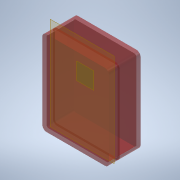
# Autodesk Inventor part: bottom
Saved by Autodesk Inventor 2020 (Build 240168000, 168)
## iProperties
Created: 2019-03-25
Part Number: bottom
Material: Generic
Document SubType Name: Modeling
Designer: erwin
Density: 1 g/cm^3
Appearance: Default
Author: erwin
Autodesk Inventor part; units mm, degrees
ref_plane "YZ Plane" through (0, 0, 0) normal (1, 0, 0) x (0, 1, 0)
ref_plane "XZ Plane" through (0, 0, 0) normal (0, 1, 0) x (-1, 0, 0)
ref_plane "Work Plane3" through (-33.721, -16.0631, -8.3772) normal (0, 0, -1) x (-1, 0, 0)
sketch "Sketch2" plane through (-33.721, -16.0631, -8.3772) normal (0, 0, -1) x (-1, 0, 0)
  line L0 (3.351, 52.725) -> (-59.649, 52.725)
  line L1 (-59.649, 52.725) -> (-59.649, -27.275)
  line L2 (-59.649, -27.275) -> (3.351, -27.275)
  line L3 (3.351, -27.275) -> (3.351, 52.725)
  line L4 (3.351, 52.725) -> (-59.649, -27.275) construction
  line L5 (-59.649, 52.725) -> (3.351, -27.275) construction
  line L6 (-25.524, -24.775) -> (-3.524, -24.775) projected
  line L7 (-0.024, 32.975) -> (-0.024, 14.6) projected
  line L8 (-56.274, -10.275) -> (-56.274, 32.975)
  line L9 (-3.524, 50.225) -> (-25.524, 50.225) projected
  line L10 (-1.524, 34.475) -> (-56.274, 34.475) projected
  line L11 (-56.274, -11.775) -> (-56.274, 34.475) projected
  line L12 (-56.274, -11.775) -> (-1.524, -11.775) projected
  line L13 (-1.524, -11.775) -> (-1.1358, -11.7239) projected
  line L14 (-0.774, -11.574) -> (-1.1358, -11.7239) projected
  line L15 (-0.4633, -11.3357) -> (-0.774, -11.574) projected
  line L16 (-0.4633, -11.3357) -> (-0.225, -11.025) projected
  line L17 (-0.0751, -10.6632) -> (-0.225, -11.025) projected
  line L18 (-0.024, -10.275) -> (-0.0751, -10.6632) projected
  line L19 (-0.024, 0) -> (-0.024, -10.275) projected
  line L20 (-0.024, 0) -> (-14.65, 0) projected
  line L21 (-14.65, 14.6) -> (-14.65, 0) projected
  line L22 (-0.024, 14.6) -> (-14.65, 14.6) projected
  line L23 (-0.024, 32.975) -> (-0.024, 14.6) projected
  line L24 (-0.024, 32.975) -> (-0.0751, 33.3632) projected
  line L25 (-0.0751, 33.3632) -> (-0.225, 33.725) projected
  line L26 (-0.225, 33.725) -> (-0.4633, 34.0357) projected
  line L27 (-0.774, 34.274) -> (-0.4633, 34.0357) projected
  line L28 (-1.1358, 34.4239) -> (-0.774, 34.274) projected
  line L29 (-1.1358, 34.4239) -> (-1.524, 34.475) projected
  line L30 (-46.714, -1.95) -> (-47.364, -1.95) projected
  line L31 (-46.714, -1.95) -> (-46.714, -2.6) projected
  line L32 (-47.364, -2.6) -> (-46.714, -2.6) projected
  line L33 (-47.364, -2.6) -> (-47.364, -1.95) projected
  line L34 (-37.794, -7.64) -> (-38.444, -7.64) projected
  line L35 (-37.794, -8.29) -> (-37.794, -7.64) projected
  line L36 (-38.444, -8.29) -> (-37.794, -8.29) projected
  line L37 (-38.444, -8.29) -> (-38.444, -7.64) projected
  line L38 (-2.8885, -10.3772) -> (-3.149, -10.4) projected
  line L39 (-3.4095, -10.3772) -> (-3.149, -10.4) projected
  line L40 (-3.662, -10.3095) -> (-3.4095, -10.3772) projected
  line L41 (-3.899, -10.199) -> (-3.662, -10.3095) projected
  line L42 (-3.899, -10.199) -> (-4.1132, -10.0491) projected
  line L43 (-4.1132, -10.0491) -> (-4.2981, -9.8642) projected
  line L44 (-4.2981, -9.8642) -> (-4.448, -9.65) projected
  line L45 (-4.5585, -9.413) -> (-4.448, -9.65) projected
  line L46 (-4.5585, -9.413) -> (-4.6262, -9.1605) projected
  line L47 (-4.6262, -9.1605) -> (-4.649, -8.9) projected
  line L48 (-4.649, -8.9) -> (-4.6262, -8.6395) projected
  line L49 (-4.5585, -8.387) -> (-4.6262, -8.6395) projected
  line L50 (-4.5585, -8.387) -> (-4.448, -8.15) projected
  line L51 (-4.448, -8.15) -> (-4.2981, -7.9358) projected
  line L52 (-4.2981, -7.9358) -> (-4.1132, -7.7509) projected
  line L53 (-3.899, -7.601) -> (-4.1132, -7.7509) projected
  line L54 (-3.662, -7.4905) -> (-3.899, -7.601) projected
  line L55 (-3.662, -7.4905) -> (-3.4095, -7.4228) projected
  line L56 (-3.4095, -7.4228) -> (-3.149, -7.4) projected
  line L57 (-2.8885, -7.4228) -> (-3.149, -7.4) projected
  line L58 (-2.636, -7.4905) -> (-2.8885, -7.4228) projected
  line L59 (-2.399, -7.601) -> (-2.636, -7.4905) projected
  line L60 (-2.399, -7.601) -> (-2.1848, -7.7509) projected
  line L61 (-1.9999, -7.9358) -> (-2.1848, -7.7509) projected
  line L62 (-1.85, -8.15) -> (-1.9999, -7.9358) projected
  line L63 (-1.85, -8.15) -> (-1.7395, -8.387) projected
  line L64 (-1.7395, -8.387) -> (-1.6718, -8.6395) projected
  line L65 (-1.6718, -8.6395) -> (-1.649, -8.9) projected
  line L66 (-1.649, -8.9) -> (-1.6718, -9.1605) projected
  line L67 (-1.7395, -9.413) -> (-1.6718, -9.1605) projected
  line L68 (-1.7395, -9.413) -> (-1.85, -9.65) projected
  line L69 (-1.9999, -9.8642) -> (-1.85, -9.65) projected
  line L70 (-1.9999, -9.8642) -> (-2.1848, -10.0491) projected
  line L71 (-2.399, -10.199) -> (-2.1848, -10.0491) projected
  line L72 (-2.636, -10.3095) -> (-2.399, -10.199) projected
  line L73 (-2.636, -10.3095) -> (-2.8885, -10.3772) projected
  line L74 (-7.964, -8.29) -> (-7.314, -8.29) projected
  line L75 (-7.964, -8.29) -> (-7.964, -7.64) projected
  line L76 (-7.964, -7.64) -> (-7.314, -7.64) projected
  line L77 (-7.314, -7.64) -> (-7.314, -8.29) projected
  line L78 (-10.504, -10.83) -> (-9.854, -10.83) projected
  line L79 (-10.504, -10.18) -> (-10.504, -10.83) projected
  line L80 (-10.504, -10.18) -> (-9.854, -10.18) projected
  line L81 (-9.854, -10.18) -> (-9.854, -10.83) projected
  line L82 (-15.584, -10.83) -> (-14.934, -10.83) projected
  line L83 (-15.584, -10.18) -> (-15.584, -10.83) projected
  line L84 (-14.934, -10.18) -> (-15.584, -10.18) projected
  line L85 (-14.934, -10.18) -> (-14.934, -10.83) projected
  line L86 (-15.584, -8.29) -> (-14.934, -8.29) projected
  line L87 (-15.584, -7.64) -> (-15.584, -8.29) projected
  line L88 (-15.584, -7.64) -> (-14.934, -7.64) projected
  line L89 (-14.934, -7.64) -> (-14.934, -8.29) projected
  line L90 (-17.474, -7.64) -> (-17.474, -8.29) projected
  line L91 (-18.124, -8.29) -> (-17.474, -8.29) projected
  line L92 (-18.124, -7.64) -> (-18.124, -8.29) projected
  line L93 (-17.474, -7.64) -> (-18.124, -7.64) projected
  line L94 (-20.014, -7.64) -> (-20.014, -8.29) projected
  line L95 (-20.664, -8.29) -> (-20.014, -8.29) projected
  line L96 (-20.664, -7.64) -> (-20.664, -8.29) projected
  line L97 (-20.014, -7.64) -> (-20.664, -7.64) projected
  line L98 (-22.554, -7.64) -> (-22.554, -8.29) projected
  line L99 (-23.204, -8.29) -> (-22.554, -8.29) projected
  line L100 (-23.204, -7.64) -> (-23.204, -8.29) projected
  line L101 (-22.554, -7.64) -> (-23.204, -7.64) projected
  line L102 (-25.094, -7.64) -> (-25.094, -8.29) projected
  line L103 (-25.744, -8.29) -> (-25.094, -8.29) projected
  line L104 (-25.744, -7.64) -> (-25.744, -8.29) projected
  line L105 (-25.094, -7.64) -> (-25.744, -7.64) projected
  line L106 (-27.634, -7.64) -> (-27.634, -8.29) projected
  line L107 (-28.284, -8.29) -> (-27.634, -8.29) projected
  line L108 (-28.284, -8.29) -> (-28.284, -7.64) projected
  line L109 (-27.634, -7.64) -> (-28.284, -7.64) projected
  line L110 (-30.824, -10.83) -> (-30.174, -10.83) projected
  line L111 (-30.824, -10.18) -> (-30.824, -10.83) projected
  line L112 (-30.174, -10.18) -> (-30.824, -10.18) projected
  line L113 (-30.174, -10.18) -> (-30.174, -10.83) projected
  line L114 (-33.364, -10.83) -> (-32.714, -10.83) projected
  line L115 (-33.364, -10.18) -> (-33.364, -10.83) projected
  line L116 (-32.714, -10.18) -> (-33.364, -10.18) projected
  line L117 (-32.714, -10.18) -> (-32.714, -10.83) projected
  line L118 (-35.904, -10.83) -> (-35.254, -10.83) projected
  line L119 (-35.904, -10.18) -> (-35.904, -10.83) projected
  line L120 (-35.254, -10.18) -> (-35.904, -10.18) projected
  line L121 (-35.254, -10.18) -> (-35.254, -10.83) projected
  line L122 (-38.444, -10.83) -> (-37.794, -10.83) projected
  line L123 (-38.444, -10.18) -> (-38.444, -10.83) projected
  line L124 (-37.794, -10.18) -> (-38.444, -10.18) projected
  line L125 (-37.794, -10.18) -> (-37.794, -10.83) projected
  line L126 (-40.984, -10.83) -> (-40.334, -10.83) projected
  line L127 (-40.984, -10.18) -> (-40.984, -10.83) projected
  line L128 (-40.334, -10.18) -> (-40.984, -10.18) projected
  line L129 (-40.334, -10.18) -> (-40.334, -10.83) projected
  line L130 (-35.254, -7.64) -> (-35.254, -8.29) projected
  line L131 (-35.904, -8.29) -> (-35.254, -8.29) projected
  line L132 (-35.904, -8.29) -> (-35.904, -7.64) projected
  line L133 (-35.254, -7.64) -> (-35.904, -7.64) projected
  line L134 (-32.714, -7.64) -> (-32.714, -8.29) projected
  line L135 (-33.364, -8.29) -> (-32.714, -8.29) projected
  line L136 (-33.364, -8.29) -> (-33.364, -7.64) projected
  line L137 (-32.714, -7.64) -> (-33.364, -7.64) projected
  line L138 (-30.174, -7.64) -> (-30.174, -8.29) projected
  line L139 (-30.824, -8.29) -> (-30.174, -8.29) projected
  line L140 (-30.824, -8.29) -> (-30.824, -7.64) projected
  line L141 (-30.174, -7.64) -> (-30.824, -7.64) projected
  line L142 (-28.284, -10.83) -> (-27.634, -10.83) projected
  line L143 (-28.284, -10.18) -> (-28.284, -10.83) projected
  line L144 (-27.634, -10.18) -> (-28.284, -10.18) projected
  line L145 (-27.634, -10.18) -> (-27.634, -10.83) projected
  line L146 (-25.744, -10.83) -> (-25.094, -10.83) projected
  line L147 (-25.744, -10.18) -> (-25.744, -10.83) projected
  line L148 (-25.094, -10.18) -> (-25.744, -10.18) projected
  line L149 (-25.094, -10.18) -> (-25.094, -10.83) projected
  line L150 (-23.204, -10.83) -> (-22.554, -10.83) projected
  line L151 (-23.204, -10.18) -> (-23.204, -10.83) projected
  line L152 (-22.554, -10.18) -> (-23.204, -10.18) projected
  line L153 (-22.554, -10.18) -> (-22.554, -10.83) projected
  line L154 (-20.664, -10.83) -> (-20.014, -10.83) projected
  line L155 (-20.664, -10.18) -> (-20.664, -10.83) projected
  line L156 (-20.014, -10.18) -> (-20.664, -10.18) projected
  line L157 (-20.014, -10.18) -> (-20.014, -10.83) projected
  line L158 (-10.504, -8.29) -> (-9.854, -8.29) projected
  line L159 (-10.504, -8.29) -> (-10.504, -7.64) projected
  line L160 (-10.504, -7.64) -> (-9.854, -7.64) projected
  line L161 (-9.854, -7.64) -> (-9.854, -8.29) projected
  line L162 (-12.394, -8.29) -> (-12.394, -7.64) projected
  line L163 (-13.044, -8.29) -> (-12.394, -8.29) projected
  line L164 (-13.044, -8.29) -> (-13.044, -7.64) projected
  line L165 (-13.044, -7.64) -> (-12.394, -7.64) projected
  line L166 (-18.124, -10.83) -> (-17.474, -10.83) projected
  line L167 (-18.124, -10.18) -> (-18.124, -10.83) projected
  line L168 (-17.474, -10.18) -> (-18.124, -10.18) projected
  line L169 (-17.474, -10.18) -> (-17.474, -10.83) projected
  line L170 (-13.044, -10.83) -> (-12.394, -10.83) projected
  line L171 (-13.044, -10.18) -> (-13.044, -10.83) projected
  line L172 (-12.394, -10.18) -> (-13.044, -10.18) projected
  line L173 (-12.394, -10.18) -> (-12.394, -10.83) projected
  line L174 (-7.964, -10.83) -> (-7.314, -10.83) projected
  line L175 (-7.964, -10.18) -> (-7.964, -10.83) projected
  line L176 (-7.964, -10.18) -> (-7.314, -10.18) projected
  line L177 (-7.314, -10.18) -> (-7.314, -10.83) projected
  line L178 (-40.334, -8.29) -> (-40.334, -7.64) projected
  line L179 (-40.984, -8.29) -> (-40.334, -8.29) projected
  line L180 (-40.984, -8.29) -> (-40.984, -7.64) projected
  line L181 (-40.984, -7.64) -> (-40.334, -7.64) projected
  line L182 (-44.174, -2.6) -> (-44.174, -1.95) projected
  line L183 (-44.824, -2.6) -> (-44.174, -2.6) projected
  line L184 (-44.824, -1.95) -> (-44.824, -2.6) projected
  line L185 (-44.824, -1.95) -> (-44.174, -1.95) projected
  line L186 (-37.794, 32.88) -> (-37.794, 33.53) projected
  line L187 (-37.794, 32.88) -> (-38.444, 32.88) projected
  line L188 (-38.444, 32.88) -> (-38.444, 33.53) projected
  line L189 (-38.444, 33.53) -> (-37.794, 33.53) projected
  line L190 (-35.254, 32.88) -> (-35.254, 33.53) projected
  line L191 (-35.254, 32.88) -> (-35.904, 32.88) projected
  line L192 (-35.904, 32.88) -> (-35.904, 33.53) projected
  line L193 (-35.904, 33.53) -> (-35.254, 33.53) projected
  line L194 (-32.714, 32.88) -> (-32.714, 33.53) projected
  line L195 (-32.714, 32.88) -> (-33.364, 32.88) projected
  line L196 (-33.364, 32.88) -> (-33.364, 33.53) projected
  line L197 (-33.364, 33.53) -> (-32.714, 33.53) projected
  line L198 (-30.174, 32.88) -> (-30.174, 33.53) projected
  line L199 (-30.174, 32.88) -> (-30.824, 32.88) projected
  line L200 (-30.824, 32.88) -> (-30.824, 33.53) projected
  line L201 (-30.824, 33.53) -> (-30.174, 33.53) projected
  line L202 (-27.634, 32.88) -> (-27.634, 33.53) projected
  line L203 (-27.634, 32.88) -> (-28.284, 32.88) projected
  line L204 (-28.284, 32.88) -> (-28.284, 33.53) projected
  line L205 (-28.284, 33.53) -> (-27.634, 33.53) projected
  line L206 (-25.094, 32.88) -> (-25.094, 33.53) projected
  line L207 (-25.744, 32.88) -> (-25.094, 32.88) projected
  line L208 (-25.744, 32.88) -> (-25.744, 33.53) projected
  line L209 (-25.744, 33.53) -> (-25.094, 33.53) projected
  line L210 (-22.554, 32.88) -> (-22.554, 33.53) projected
  line L211 (-23.204, 32.88) -> (-22.554, 32.88) projected
  line L212 (-23.204, 32.88) -> (-23.204, 33.53) projected
  line L213 (-23.204, 33.53) -> (-22.554, 33.53) projected
  line L214 (-20.014, 32.88) -> (-20.014, 33.53) projected
  line L215 (-20.664, 32.88) -> (-20.014, 32.88) projected
  line L216 (-20.664, 32.88) -> (-20.664, 33.53) projected
  line L217 (-20.664, 33.53) -> (-20.014, 33.53) projected
  line L218 (-17.474, 32.88) -> (-17.474, 33.53) projected
  line L219 (-18.124, 32.88) -> (-17.474, 32.88) projected
  line L220 (-18.124, 32.88) -> (-18.124, 33.53) projected
  line L221 (-18.124, 33.53) -> (-17.474, 33.53) projected
  line L222 (-14.934, 32.88) -> (-14.934, 33.53) projected
  line L223 (-15.584, 32.88) -> (-14.934, 32.88) projected
  line L224 (-15.584, 32.88) -> (-15.584, 33.53) projected
  line L225 (-15.584, 33.53) -> (-14.934, 33.53) projected
  line L226 (-12.394, 32.88) -> (-12.394, 33.53) projected
  line L227 (-12.394, 32.88) -> (-13.044, 32.88) projected
  line L228 (-13.044, 32.88) -> (-13.044, 33.53) projected
  line L229 (-12.394, 33.53) -> (-13.044, 33.53) projected
  line L230 (-9.854, 32.88) -> (-9.854, 33.53) projected
  line L231 (-10.504, 32.88) -> (-9.854, 32.88) projected
  line L232 (-10.504, 32.88) -> (-10.504, 33.53) projected
  line L233 (-9.854, 33.53) -> (-10.504, 33.53) projected
  line L234 (-7.314, 32.88) -> (-7.314, 33.53) projected
  line L235 (-7.964, 32.88) -> (-7.314, 32.88) projected
  line L236 (-7.964, 32.88) -> (-7.964, 33.53) projected
  line L237 (-7.964, 33.53) -> (-7.314, 33.53) projected
  line L238 (-1.6718, 31.8605) -> (-1.7395, 32.113) projected
  line L239 (-1.6718, 31.8605) -> (-1.649, 31.6) projected
  line L240 (-1.649, 31.6) -> (-1.6718, 31.3395) projected
  line L241 (-1.7395, 31.087) -> (-1.6718, 31.3395) projected
  line L242 (-1.7395, 31.087) -> (-1.85, 30.85) projected
  line L243 (-1.85, 30.85) -> (-1.9999, 30.6358) projected
  line L244 (-2.1848, 30.4509) -> (-1.9999, 30.6358) projected
  line L245 (-2.1848, 30.4509) -> (-2.399, 30.301) projected
  line L246 (-2.636, 30.1905) -> (-2.399, 30.301) projected
  line L247 (-2.8885, 30.1228) -> (-2.636, 30.1905) projected
  line L248 (-3.149, 30.1) -> (-2.8885, 30.1228) projected
  line L249 (-3.4095, 30.1228) -> (-3.149, 30.1) projected
  line L250 (-3.4095, 30.1228) -> (-3.662, 30.1905) projected
  line L251 (-3.899, 30.301) -> (-3.662, 30.1905) projected
  line L252 (-4.1132, 30.4509) -> (-3.899, 30.301) projected
  line L253 (-4.1132, 30.4509) -> (-4.2981, 30.6358) projected
  line L254 (-4.448, 30.85) -> (-4.2981, 30.6358) projected
  line L255 (-4.448, 30.85) -> (-4.5585, 31.087) projected
  line L256 (-4.5585, 31.087) -> (-4.6262, 31.3395) projected
  line L257 (-4.649, 31.6) -> (-4.6262, 31.3395) projected
  line L258 (-4.649, 31.6) -> (-4.6262, 31.8605) projected
  line L259 (-4.6262, 31.8605) -> (-4.5585, 32.113) projected
  line L260 (-4.5585, 32.113) -> (-4.448, 32.35) projected
  line L261 (-4.2981, 32.5642) -> (-4.448, 32.35) projected
  line L262 (-4.2981, 32.5642) -> (-4.1132, 32.7491) projected
  line L263 (-4.1132, 32.7491) -> (-3.899, 32.899) projected
  line L264 (-3.662, 33.0095) -> (-3.899, 32.899) projected
  line L265 (-3.4095, 33.0772) -> (-3.662, 33.0095) projected
  line L266 (-3.149, 33.1) -> (-3.4095, 33.0772) projected
  line L267 (-3.149, 33.1) -> (-2.8885, 33.0772) projected
  line L268 (-2.636, 33.0095) -> (-2.8885, 33.0772) projected
  line L269 (-2.399, 32.899) -> (-2.636, 33.0095) projected
  line L270 (-2.1848, 32.7491) -> (-2.399, 32.899) projected
  line L271 (-2.1848, 32.7491) -> (-1.9999, 32.5642) projected
  line L272 (-1.9999, 32.5642) -> (-1.85, 32.35) projected
  line L273 (-1.85, 32.35) -> (-1.7395, 32.113) projected
  line L274 (-44.399, 30.301) -> (-44.1848, 30.4509) projected
  line L275 (-44.636, 30.1905) -> (-44.399, 30.301) projected
  line L276 (-44.636, 30.1905) -> (-44.8885, 30.1228) projected
  line L277 (-45.149, 30.1) -> (-44.8885, 30.1228) projected
  line L278 (-45.4095, 30.1228) -> (-45.149, 30.1) projected
  line L279 (-45.4095, 30.1228) -> (-45.662, 30.1905) projected
  line L280 (-45.662, 30.1905) -> (-45.899, 30.301) projected
  line L281 (-45.899, 30.301) -> (-46.1132, 30.4509) projected
  line L282 (-46.1132, 30.4509) -> (-46.2981, 30.6358) projected
  line L283 (-46.2981, 30.6358) -> (-46.448, 30.85) projected
  line L284 (-46.448, 30.85) -> (-46.5585, 31.087) projected
  line L285 (-46.6262, 31.3395) -> (-46.5585, 31.087) projected
  line L286 (-46.649, 31.6) -> (-46.6262, 31.3395) projected
  line L287 (-46.649, 31.6) -> (-46.6262, 31.8605) projected
  line L288 (-46.6262, 31.8605) -> (-46.5585, 32.113) projected
  line L289 (-46.5585, 32.113) -> (-46.448, 32.35) projected
  line L290 (-46.448, 32.35) -> (-46.2981, 32.5642) projected
  line L291 (-46.1132, 32.7491) -> (-46.2981, 32.5642) projected
  line L292 (-45.899, 32.899) -> (-46.1132, 32.7491) projected
  line L293 (-45.899, 32.899) -> (-45.662, 33.0095) projected
  line L294 (-45.4095, 33.0772) -> (-45.662, 33.0095) projected
  line L295 (-45.149, 33.1) -> (-45.4095, 33.0772) projected
  line L296 (-44.8885, 33.0772) -> (-45.149, 33.1) projected
  line L297 (-44.8885, 33.0772) -> (-44.636, 33.0095) projected
  line L298 (-44.399, 32.899) -> (-44.636, 33.0095) projected
  line L299 (-44.399, 32.899) -> (-44.1848, 32.7491) projected
  line L300 (-43.9999, 32.5642) -> (-44.1848, 32.7491) projected
  line L301 (-43.9999, 32.5642) -> (-43.85, 32.35) projected
  line L302 (-43.85, 32.35) -> (-43.7395, 32.113) projected
  line L303 (-43.7395, 32.113) -> (-43.6718, 31.8605) projected
  line L304 (-43.6718, 31.8605) -> (-43.649, 31.6) projected
  line L305 (-43.649, 31.6) -> (-43.6718, 31.3395) projected
  line L306 (-43.6718, 31.3395) -> (-43.7395, 31.087) projected
  line L307 (-43.85, 30.85) -> (-43.7395, 31.087) projected
  line L308 (-43.85, 30.85) -> (-43.9999, 30.6358) projected
  line L309 (-43.9999, 30.6358) -> (-44.1848, 30.4509) projected
  line L310 (-40.984, 32.88) -> (-40.984, 33.53) projected
  line L311 (-40.984, 33.53) -> (-40.334, 33.53) projected
  line L312 (-40.334, 32.88) -> (-40.334, 33.53) projected
  line L313 (-40.334, 32.88) -> (-40.984, 32.88) projected
  line L314 (-41.634, -1.95) -> (-41.634, -2.6) projected
  line L315 (-41.634, -2.6) -> (-42.284, -2.6) projected
  line L316 (-42.284, -2.6) -> (-42.284, -1.95) projected
  line L317 (-41.634, -1.95) -> (-42.284, -1.95) projected
  line L318 (-43.7395, -8.387) -> (-43.6718, -8.6395) projected
  line L319 (-43.6718, -8.6395) -> (-43.649, -8.9) projected
  line L320 (-43.649, -8.9) -> (-43.6718, -9.1605) projected
  line L321 (-43.6718, -9.1605) -> (-43.7395, -9.413) projected
  line L322 (-43.85, -9.65) -> (-43.7395, -9.413) projected
  line L323 (-43.85, -9.65) -> (-43.9999, -9.8642) projected
  line L324 (-44.1848, -10.0491) -> (-43.9999, -9.8642) projected
  line L325 (-44.399, -10.199) -> (-44.1848, -10.0491) projected
  line L326 (-44.636, -10.3095) -> (-44.399, -10.199) projected
  line L327 (-44.8885, -10.3772) -> (-44.636, -10.3095) projected
  line L328 (-45.149, -10.4) -> (-44.8885, -10.3772) projected
  line L329 (-45.4095, -10.3772) -> (-45.149, -10.4) projected
  line L330 (-45.4095, -10.3772) -> (-45.662, -10.3095) projected
  line L331 (-45.662, -10.3095) -> (-45.899, -10.199) projected
  line L332 (-46.1132, -10.0491) -> (-45.899, -10.199) projected
  line L333 (-46.2981, -9.8642) -> (-46.1132, -10.0491) projected
  line L334 (-46.2981, -9.8642) -> (-46.448, -9.65) projected
  line L335 (-46.448, -9.65) -> (-46.5585, -9.413) projected
  line L336 (-46.6262, -9.1605) -> (-46.5585, -9.413) projected
  line L337 (-46.649, -8.9) -> (-46.6262, -9.1605) projected
  line L338 (-46.649, -8.9) -> (-46.6262, -8.6395) projected
  line L339 (-46.6262, -8.6395) -> (-46.5585, -8.387) projected
  line L340 (-46.5585, -8.387) -> (-46.448, -8.15) projected
  line L341 (-46.448, -8.15) -> (-46.2981, -7.9358) projected
  line L342 (-46.1132, -7.7509) -> (-46.2981, -7.9358) projected
  line L343 (-45.899, -7.601) -> (-46.1132, -7.7509) projected
  line L344 (-45.899, -7.601) -> (-45.662, -7.4905) projected
  line L345 (-45.4095, -7.4228) -> (-45.662, -7.4905) projected
  line L346 (-45.149, -7.4) -> (-45.4095, -7.4228) projected
  line L347 (-44.8885, -7.4228) -> (-45.149, -7.4) projected
  line L348 (-44.8885, -7.4228) -> (-44.636, -7.4905) projected
  line L349 (-44.399, -7.601) -> (-44.636, -7.4905) projected
  line L350 (-44.399, -7.601) -> (-44.1848, -7.7509) projected
  line L351 (-43.9999, -7.9358) -> (-44.1848, -7.7509) projected
  line L352 (-43.9999, -7.9358) -> (-43.85, -8.15) projected
  line L353 (-43.85, -8.15) -> (-43.7395, -8.387) projected
  point P0 (-33.721, 16.0631)
  point P1 (-28.149, 12.725)
  dimension "d2" = 63
  dimension "d3" = 80
  dimension "d4" = 2.5
  dimension "d5" = 3.375
  dimension "d6" = 3.375
  dimension "d7" = 2.5
  constraints: 14 end point, 2 midpoint, 2 parallel, 1 horizontal, 1 perpendicular, 1 vertical
  measures "d2" distance of L2.end L1.end
  measures "d3" distance of L1.end L0.end
  measures "d4" distance between parallel lines of L0 L9
  measures "d5" distance between parallel lines of L3 L7
  measures "d6" distance between parallel lines of L1 L8
  measures "d7" distance between parallel lines of L2 L6
ref_plane "Work Plane4" through (-28.697, -42.3381, 21.3728) normal (0, 0, 1) x (1, 0, 0)
extrude "Extrusion1" add sketch "Sketch2" against normal up to surface (29.75 mm away) contours L3 L2 L1 L0 | L7 L22 L21 L20 L19 L18 L17 L16 L15 L14 L13 L12 L11 L8 L10 L29 L28 L27 L26 L25 L24 | L31 L32 L33 L30 | L35 L36 L37 L34 | L38 L39 L40 L41 L42 L43 L44 L45 L46 L47 L48 L49 L50 L51 L52 L53 L54 L55 L56 L57 L58 L59 L60 L61 L62 L63 L64 L65 L66 L67 L68 L69 L70 L71 L72 L73 | L75 L76 L77 L74 | L79 L80 L81 L78 | L83 L84 L85 L82 | L87 L88 L89 L86 | L90 L91 L92 L93 | L94 L95 L96 L97 | L98 L99 L100 L101 | L102 L103 L104 L105 | L106 L107 L108 L109 | L111 L112 L113 L110 | L115 L116 L117 L114 | L119 L120 L121 L118 | L123 L124 L125 L122 | L127 L128 L129 L126 | L130 L131 L132 L133 | L134 L135 L136 L137 | L138 L139 L140 L141 | L143 L144 L145 L142 | L147 L148 L149 L146 | L151 L152 L153 L150 | L155 L156 L157 L154 | L159 L160 L161 L158 | L163 L164 L165 L162 | L167 L168 L169 L166 | L171 L172 L173 L170 | L175 L176 L177 L174 | L179 L180 L181 L178 | L183 L184 L185 L182 | L187 L188 L189 L186 | L191 L192 L193 L190 | L195 L196 L197 L194 | L199 L200 L201 L198 | L203 L204 L205 L202 | L207 L208 L209 L206 | L211 L212 L213 L210 | L215 L216 L217 L214 | L219 L220 L221 L218 | L223 L224 L225 L222 | L227 L228 L229 L226 | L231 L232 L233 L230 | L235 L236 L237 L234 | L239 L240 L241 L242 L243 L244 L245 L246 L247 L248 L249 L250 L251 L252 L253 L254 L255 L256 L257 L258 L259 L260 L261 L262 L263 L264 L265 L266 L267 L268 L269 L270 L271 L272 L273 L238 | L275 L276 L277 L278 L279 L280 L281 L282 L283 L284 L285 L286 L287 L288 L289 L290 L291 L292 L293 L294 L295 L296 L297 L298 L299 L300 L301 L302 L303 L304 L305 L306 L307 L308 L309 L274 | L310 L311 L312 L313 | L314 L315 L316 L317 | L318 L319 L320 L321 L322 L323 L324 L325 L326 L327 L328 L329 L330 L331 L332 L333 L334 L335 L336 L337 L338 L339 L340 L341 L342 L343 L344 L345 L346 L347 L348 L349 L350 L351 L352 L353
fillet "Fillet1" radius 4 4 edges at (-37.072, -43.3381, 6.4978) (25.928, -43.3381, 6.4978) (25.928, 36.6619, 6.4978) (-37.072, 36.6619, 6.4978)
shell "Shell1" thickness 2 removed faces 0
ref_plane "Work Plane5" through (-8.197, -40.8381, 11.3728) normal (0, 0, 1) x (1, 0, 0)
split body "Split1" result two bodies by plane through (-8.197, -40.8381, 11.3728) normal (0, 0, 1) first body at (4.928, 8.6619, 20.8728)
equation "\"d6\" = d5"
equation "\"d7\" = d4"
body "Solid2"
body "Solid3"
